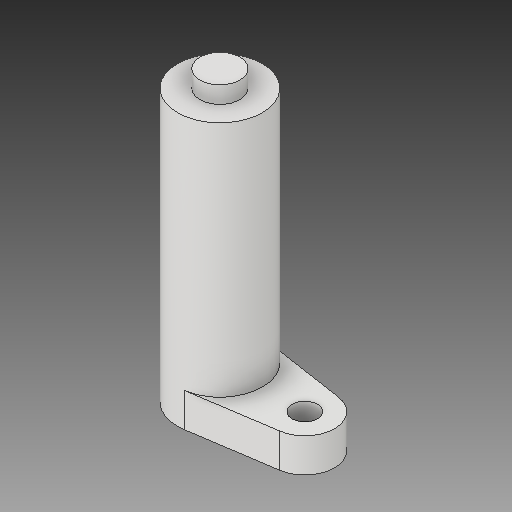
# Autodesk Inventor part: Pok Mk3 Yaw Motor Support Min
Saved by Autodesk Inventor 2018.2 (Build 222227000, 227)
## iProperties
Created: 2018-02-27
Part Number: Pok Mk3 Yaw Motor Support Min
Material: ABS Plastic
Document SubType Name: Modeling
Designer: Moochster
Density: 1.06 g/cm^3
Appearance: Smooth - White
Mass: 2.95043 g
Surface Area: 14.094 cm^2
Volume: 2.78342 cm^3
Author: Moochster
Autodesk Inventor part; units mm, degrees
ref_plane "XZ Plane" through (0, 0, 0) normal (0, 1, 0) x (-1, 0, 0)
sketch "Sketch1" plane through (0, 0, 0) normal (0, 1, 0) x (-1, 0, 0)
  circle A0 centre (0, 0) radius 2.35
  circle A1 centre (0, 0) radius 5
  circle A2 centre (-10, 0) radius 1.5
  line L0 (-0.75, 4.9434) -> (-10.525, 3.4604)
  arc A3 (-10.525, 3.4604) -> (-10.525, -3.4604) centre (-10, 0) ccw
  line L1 (-10.525, -3.4604) -> (-0.75, -4.9434)
  dimension "d0" = 4.7
  dimension "d1" = 10
  dimension "d2" = 3
  dimension "d3" = 10
  dimension "d4" = 2
  constraints: 4 centre point, 4 end point, 4 point on circle, 4 tangent, 3 coincident, 1 concentric, 1 horizontal alignment
  measures "d0" diameter of A0
  measures "d1" diameter of A1
  measures "d2" diameter of A2
  measures "d3" distance of point (0, 0) A2.centre
  measures "d4" radial gap between concentric circles of A2 A3
extrude "Extrusion1" add sketch "Sketch1" against normal blind 2 and the other way blind 2 contours A0 | A1 | A1 L1 A3 L0
extrude "Extrusion2" add sketch "Sketch1" along normal blind 30 contours A1
extrude "Extrusion3" add sketch "Sketch1" along normal blind 32 contours A0
ref_plane "Work Plane1" through (-5, 0, 0) normal (1, 0, 0) x (0, 1, 0)
ref_plane "Work Plane2" through (-7, 0, 0) normal (1, 0, 0) x (0, 1, 0)
sketch "Sketch2" plane through (-7, 0, 0) normal (1, 0, 0) x (0, 1, 0)
  line L0 (30, -15) -> (-2, -15)
  line L1 (-2, 15) -> (30, 15)
  line L2 (30, 15) -> (30, -15)
  line L3 (30, -5) -> (30, 5) projected
  line L4 (-2, -4.9434) -> (2, -4.9434) projected
  line L5 (-2, 4.9434) -> (-2, -4.9434) projected
  line L6 (2, 4.9434) -> (-2, 4.9434) projected
  line L7 (2, -4.9434) -> (2, 4.9434) projected
  line L8 (-2, -15) -> (-2, 15)
  point P0 (0, 0)
  dimension "d11" = 30
  dimension "d12" = 15
  constraints: 8 end point, 1 horizontal, 1 parallel, 1 vertical, 1 vertical alignment
  measures "d11" distance between parallel lines of L0 L1
  measures "d12" distance from line of point (0, 0) L1
sketch "Sketch3" plane through (-7, 0, 0) normal (-1, 0, 0) x (0, 0, 1)
  line L0 (-10, 22.6542) -> (10, 22.6542) construction
  line L1 (10, 22.6542) -> (10, 2.6542) construction
  line L2 (10, 2.6542) -> (-10, 2.6542) construction
  line L3 (-10, 2.6542) -> (-10, 22.6542) construction
  line L4 (15, -2) -> (15, 30) construction
  line L5 (15, 30) -> (-15, 30) construction
  line L6 (0, 0) -> (15, 0) construction
  point P0 (0, 0)
  point P1 (10, 12.6542)
  point P2 (15, 14)
  point P3 (0, 22.6542)
  point P4 (0, 30)
  dimension "d24" = 20
  dimension "d25" = 20
  constraints: 8 end point, 4 coincident, 4 midpoint, 2 parallel, 1 horizontal, 1 perpendicular, 1 vertical alignment
  measures "d24" distance of L0.end L1.end
  measures "d25" distance of L1.end L2.end
body "Solid1"
